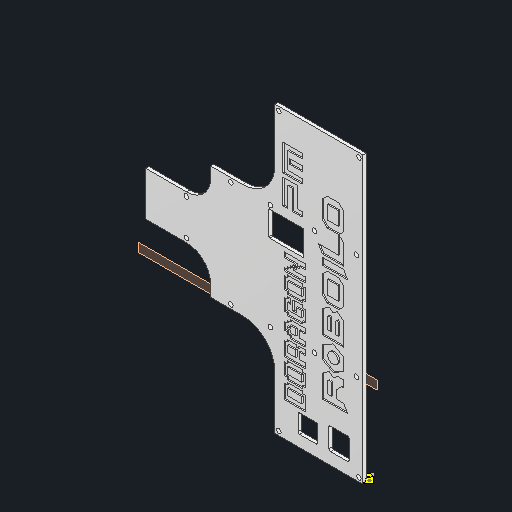
# Autodesk Inventor part: ceil
Saved by Autodesk Inventor 2023 (Build 270158000, 158)
## iProperties
Created: 2024-05-26
Part Number: ceil
Material: ABS Plastic
Document SubType Name: Modeling
Designer: szymo
Density: 1.06 g/cm^3
Appearance: Smooth - White
Mass: 27.4887 g
Surface Area: 302.13 cm^2
Volume: 25.9328 cm^3
TOTAL MASS: 0.0
Author: szymo
Autodesk Inventor part; units mm, degrees
ref_plane "YZ Plane" through (0, 0, 0) normal (1, 0, 0) x (0, 1, 0)
ref_plane "XZ Plane" through (0, 0, 0) normal (0, 1, 0) x (-1, 0, 0)
ref_plane "XY Plane" through (0, 0, 0) normal (0, 0, 1) x (1, 0, 0)
ref_plane "Work Plane1" through (-50.5, 0, 0) normal (0, 0, 1) x (1, 0, 0)
sketch "Sketch3" plane through (-50.5, 0, 0) normal (0, 0, 1) x (1, 0, 0)
  line L0 (135.5648, 0) -> (135.5648, 5.2284) projected
  line L1 (0, 5) -> (134.493, 5) projected
  line L2 (0, 0) -> (0, 5) projected
  line L3 (0, 71) -> (135.5648, 71) projected
  line L4 (0, 71) -> (0, 66) projected
  line L5 (0, 66) -> (135.5648, 66) projected
  line L6 (135.5648, 71) -> (135.5648, 66) projected
  line L7 (131.5648, 119.5) -> (134.5648, 119.5) projected
  line L8 (135.5648, 124.5) -> (135.5648, 120.5) projected
  line L9 (135.5648, 124.5) -> (51.5, 124.5) projected
  line L10 (51.5, 123.5) -> (79.5, 123.5) projected
  line L11 (80.5, 122.5) -> (80.5, 120.5) projected
  line L12 (81.5, 119.5) -> (84.5, 119.5) projected
  line L13 (85.5, 122.5) -> (85.5, 120.5) projected
  line L14 (86.5, 123.5) -> (129.5648, 123.5) projected
  line L15 (130.5648, 122.5) -> (130.5648, 120.5) projected
  line L16 (120.8148, 112) -> (120.8148, 123) projected
  line L17 (120.8148, 123) -> (94.8148, 123) projected
  line L18 (94.8148, 123) -> (94.8148, 112) projected
  line L19 (94.8148, 112) -> (120.8148, 112) projected
  line L20 (130.5648, -51.5) -> (130.5648, -49.5) projected
  line L21 (51.5, -52.5) -> (79.5, -52.5) projected
  line L22 (85.5, -51.5) -> (85.5, -49.5) projected
  line L23 (131.5648, -48.5) -> (134.5648, -48.5) projected
  line L24 (80.5, -51.5) -> (80.5, -49.5) projected
  line L25 (86.5, -52.5) -> (129.5648, -52.5) projected
  line L26 (135.5648, -53.5) -> (51.5, -53.5) projected
  line L27 (135.5648, -53.5) -> (135.5648, -49.5) projected
  line L28 (81.5, -48.5) -> (84.5, -48.5) projected
  line L29 (95.5648, -45.8) -> (95.5648, -35.2) projected
  line L30 (106.8648, -35.2) -> (95.5648, -35.2) projected
  line L31 (106.8648, -35.2) -> (106.8648, -45.8) projected
  line L32 (95.5648, -45.8) -> (106.8648, -45.8) projected
  circle A0 centre (90.4898, -49.075) radius 1.675 projected
  circle A1 centre (124.5398, -49.075) radius 1.675 projected
  line L33 (126.3648, -33.5) -> (126.3648, -45.5) projected
  line L34 (126.3648, -45.5) -> (114.7648, -45.5) projected
  line L35 (114.7648, -45.5) -> (114.7648, -33.5) projected
  line L36 (114.7648, -33.5) -> (86.8648, -33.5) projected
  line L37 (86.8648, -33.5) -> (86.8648, -52.5) projected
  line L38 (86.8648, -52.5) -> (128.0648, -52.5) projected
  line L39 (128.0648, -52.5) -> (128.0648, -33.5) projected
  line L40 (128.0648, -33.5) -> (126.3648, -33.5) projected
  line L41 (126.3648, -32.7) -> (114.7648, -32.7) projected
  line L42 (114.7648, -32.7) -> (114.7648, -45.5) projected
  line L43 (114.7648, -45.5) -> (126.3648, -45.5) projected
  line L44 (126.3648, -45.5) -> (126.3648, -32.7) projected
  line L45 (80.5, -53.5) -> (135.5648, -53.5)
  line L46 (135.5648, -53.5) -> (135.5648, 124.5)
  line L47 (135.5648, 124.5) -> (80.5, 124.5)
  line L48 (80.5, 124.5) -> (80.5, -53.5)
  line L49 (0, 22) -> (80.5, 22)
  line L50 (80.5, 22) -> (80.5, 49.5)
  line L51 (80.5, 49.5) -> (0, 49.5)
  line L52 (0, 49.5) -> (0, 22)
  line L53 (80.5, 22) -> (50.5, 22)
  line L54 (50.5, 22) -> (50.5, 0)
  line L55 (50.5, 0) -> (80.5, 0)
  line L56 (80.5, 0) -> (80.5, 22)
  line L57 (80.5, 46.5815) -> (80.5, 71)
  line L58 (80.5, 71) -> (50.5, 71)
  line L59 (50.5, 71) -> (50.5, 49.5)
  arc A2 (97.9124, 50.9) -> (98.0124, 51) centre (97.9124, 51) ccw projected
  line L60 (77.4124, 50.9) -> (97.9124, 50.9) projected
  arc A3 (77.3124, 51) -> (77.4124, 50.9) centre (77.4124, 51) ccw projected
  line L61 (77.3124, 65.5) -> (77.3124, 51) projected
  arc A4 (77.4124, 65.6) -> (77.3124, 65.5) centre (77.4124, 65.5) ccw projected
  line L62 (97.9124, 65.6) -> (77.4124, 65.6) projected
  arc A5 (98.0124, 65.5) -> (97.9124, 65.6) centre (97.9124, 65.5) ccw projected
  line L63 (98.0124, 51) -> (98.0124, 65.5) projected
  line L64 (96.2124, 63.7) -> (96.2124, 52.8) projected
  arc A6 (96.2124, 63.7) -> (95.9124, 64) centre (95.9124, 63.7) ccw projected
  line L65 (95.9124, 64) -> (95.8124, 64) projected
  line L66 (95.8124, 64) -> (95.3509, 64.55) projected
  line L67 (95.3509, 64.55) -> (94.9739, 64.55) projected
  line L68 (94.9739, 64.55) -> (94.5124, 64) projected
  line L69 (94.5124, 64) -> (90.8124, 64) projected
  line L70 (90.8124, 64) -> (90.8124, 64.35) projected
  line L71 (90.8124, 64.35) -> (89.5124, 64.35) projected
  line L72 (89.5124, 64) -> (89.5124, 64.35) projected
  line L73 (89.5124, 64) -> (85.8124, 64) projected
  line L74 (85.8124, 64) -> (85.8124, 64.35) projected
  line L75 (85.8124, 64.35) -> (84.5124, 64.35) projected
  line L76 (84.5124, 64) -> (84.5124, 64.35) projected
  line L77 (84.5124, 64) -> (80.8124, 64) projected
  line L78 (80.8124, 64) -> (80.3509, 64.55) projected
  line L79 (80.3509, 64.55) -> (79.9739, 64.55) projected
  line L80 (79.9739, 64.55) -> (79.5124, 64) projected
  line L81 (79.5124, 64) -> (79.4124, 64) projected
  arc A7 (79.4124, 64) -> (79.1124, 63.7) centre (79.4124, 63.7) ccw projected
  line L82 (79.1124, 63.7) -> (79.1124, 52.8) projected
  arc A8 (79.1124, 52.8) -> (79.4124, 52.5) centre (79.4124, 52.8) ccw projected
  line L83 (79.4124, 52.5) -> (79.5124, 52.5) projected
  line L84 (79.5124, 52.5) -> (79.9739, 51.95) projected
  line L85 (80.3509, 51.95) -> (79.9739, 51.95) projected
  line L86 (80.3509, 51.95) -> (80.8124, 52.5) projected
  line L87 (80.8124, 52.5) -> (84.5124, 52.5) projected
  line L88 (84.5124, 52.5) -> (84.5124, 52.15) projected
  line L89 (85.8124, 52.15) -> (84.5124, 52.15) projected
  line L90 (85.8124, 52.5) -> (85.8124, 52.15) projected
  line L91 (85.8124, 52.5) -> (89.5124, 52.5) projected
  line L92 (89.5124, 52.5) -> (89.5124, 52.15) projected
  line L93 (90.8124, 52.15) -> (89.5124, 52.15) projected
  line L94 (90.8124, 52.5) -> (90.8124, 52.15) projected
  line L95 (90.8124, 52.5) -> (94.5124, 52.5) projected
  line L96 (94.5124, 52.5) -> (94.9739, 51.95) projected
  line L97 (95.3509, 51.95) -> (94.9739, 51.95) projected
  line L98 (95.3509, 51.95) -> (95.8124, 52.5) projected
  line L99 (95.8124, 52.5) -> (95.9124, 52.5) projected
  arc A9 (95.9124, 52.5) -> (96.2124, 52.8) centre (95.9124, 52.8) ccw projected
  line L100 (78.1624, 55.35) -> (78.8624, 55.35) projected
  line L101 (78.8624, 55.35) -> (78.8624, 61.15) projected
  line L102 (78.1624, 61.15) -> (78.8624, 61.15) projected
  line L103 (78.1624, 61.15) -> (78.1624, 55.35) projected
  line L104 (97.1624, 61.15) -> (97.1624, 55.35) projected
  line L105 (96.4624, 61.15) -> (97.1624, 61.15) projected
  line L106 (96.4624, 55.35) -> (96.4624, 61.15) projected
  line L107 (96.4624, 55.35) -> (97.1624, 55.35) projected
  arc A10 (76.8124, 51) -> (77.4124, 50.4) centre (77.4124, 51) ccw
  line L108 (77.4124, 50.4) -> (97.9124, 50.4)
  arc A11 (97.9124, 50.4) -> (98.5124, 51) centre (97.9124, 51) ccw
  line L109 (98.5124, 51) -> (98.5124, 65.5)
  arc A12 (98.5124, 65.5) -> (97.9124, 66.1) centre (97.9124, 65.5) ccw
  line L110 (97.9124, 66.1) -> (77.4124, 66.1)
  arc A13 (77.4124, 66.1) -> (76.8124, 65.5) centre (77.4124, 65.5) ccw
  line L111 (76.8124, 65.5) -> (76.8124, 51)
  line L112 (95.0648, -34.7) -> (95.0648, -46.3)
  line L113 (95.0648, -46.3) -> (107.3648, -46.3)
  line L114 (107.3648, -46.3) -> (107.3648, -34.7)
  line L115 (107.3648, -34.7) -> (95.0648, -34.7)
  line L116 (114.2648, -45.5) -> (114.2648, -32.2)
  line L117 (114.2648, -32.2) -> (126.8648, -32.2)
  line L118 (126.8648, -32.2) -> (126.8648, -45.5)
  line L119 (126.3648, -46) -> (114.7648, -46)
  line L120 (92.8148, 110) -> (92.8148, 125)
  line L121 (92.8148, 125) -> (122.8148, 125)
  line L122 (122.8148, 125) -> (122.8148, 110)
  line L123 (122.8148, 110) -> (92.8148, 110)
  line L124 (114.2648, -45.5) -> (114.2648, -46)
  line L125 (114.2648, -46) -> (114.7648, -46)
  line L126 (126.3648, -46) -> (126.8648, -46)
  line L127 (126.8648, -46) -> (126.8648, -45.5)
  line L128 (51.5, -53.5) -> (51.5, -52.5) projected
  line L129 (51.5, 124.5) -> (51.5, 123.5) projected
  circle A14 centre (105.3205, 68.5) radius 1.75 projected
  circle A15 centre (53, 68.5) radius 1.75 projected
  circle A16 centre (77.648, 2.5) radius 1.75 projected
  circle A17 centre (131.5519, 2.5) radius 1.75 projected
  circle A18 centre (83, 122) radius 1.75 projected
  circle A19 centre (133.0648, 122) radius 1.75 projected
  arc A20 (130.5648, 120.5) -> (131.5648, 119.5) centre (131.5648, 120.5) ccw projected
  arc A21 (134.5648, 119.5) -> (135.5648, 120.5) centre (134.5648, 120.5) ccw projected
  arc A22 (80.5, 122.5) -> (79.5, 123.5) centre (79.5, 122.5) ccw projected
  arc A23 (86.5, 123.5) -> (85.5, 122.5) centre (86.5, 122.5) ccw projected
  arc A24 (130.5648, 122.5) -> (129.5648, 123.5) centre (129.5648, 122.5) ccw projected
  arc A25 (80.5, 120.5) -> (81.5, 119.5) centre (81.5, 120.5) ccw projected
  arc A26 (84.5, 119.5) -> (85.5, 120.5) centre (84.5, 120.5) ccw projected
  circle A27 centre (83, -51) radius 1.75 projected
  circle A28 centre (133.0648, -51) radius 1.75 projected
  arc A29 (131.5648, -48.5) -> (130.5648, -49.5) centre (131.5648, -49.5) ccw projected
  arc A30 (129.5648, -52.5) -> (130.5648, -51.5) centre (129.5648, -51.5) ccw projected
  arc A31 (85.5, -51.5) -> (86.5, -52.5) centre (86.5, -51.5) ccw projected
  arc A32 (79.5, -52.5) -> (80.5, -51.5) centre (79.5, -51.5) ccw projected
  arc A33 (135.5648, -49.5) -> (134.5648, -48.5) centre (134.5648, -49.5) ccw projected
  arc A34 (85.5, -49.5) -> (84.5, -48.5) centre (84.5, -49.5) ccw projected
  arc A35 (81.5, -48.5) -> (80.5, -49.5) centre (81.5, -49.5) ccw projected
  line L130 (50.5, 27) -> (0, 27) projected
  line L131 (0, 27) -> (0, 22) projected
  line L132 (50.5, 22) -> (0, 22) projected
  line L133 (50.5, 27) -> (50.5, 22) projected
  line L134 (50.5, 44.5) -> (0, 44.5) projected
  line L135 (50.5, 44.5) -> (50.5, 49.5) projected
  line L136 (50.5, 49.5) -> (0, 49.5) projected
  line L137 (0, 44.5) -> (0, 49.5) projected
  line L138 (50.5, 0) -> (40.5, 0)
  line L139 (40.5, 0) -> (40.5, 22)
  line L140 (40.5, 22) -> (50.5, 22)
  line L141 (50.5, 22) -> (50.5, 0)
  line L142 (50.5, 49.5) -> (40.5, 49.5)
  line L143 (40.5, 49.5) -> (40.5, 71)
  line L144 (40.5, 71) -> (50.5, 71)
  line L145 (50.5, 71) -> (50.5, 49.5)
  ellipse E0 centre (134.493, 7) end of major axis (136.8024, 7) minor radius 2 (134.493, 5) -> (135.5648, 5.2284) ccw projected
  circle A36 centre (25.25, 47) radius 1.75 projected
  circle A37 centre (25.25, 24.5) radius 1.75 projected
  line L146 (0, 0) -> (3.5, 0) projected
  line L147 (3.5, 0) -> (47, 0) projected
  line L148 (47, 0) -> (135.5648, 0) projected
  circle A38 centre (105.3205, 2.5) radius 1.75 projected
  circle A39 centre (53, 2.5) radius 1.75 projected
  point P0 (80.5, -49.5)
  point P1 (80.5, -52.5)
  point P2 (122.8148, 124.5)
  point P3 (92.8148, 124.5)
  point P4 (0, 44)
  point P5 (50.5, 44)
  point P6 (122.8148, 124.5)
  point P7 (122.8148, 123.5)
  point P8 (92.8148, 123.5)
  point P9 (92.8148, 124.5)
  point P10 (80.5, 123.5)
  point P11 (50.5, 66)
  point P12 (50.5, 5)
  point P13 (80.5, -52.5)
  point P14 (80.5, 66)
  point P15 (80.5, 5)
  point P16 (135.5648, 5)
  point P17 (80.5, 22)
  point P18 (50.5, 27)
  point P19 (0, 27)
  point P20 (135.5648, -49.5)
  point P21 (80.5, -49.5)
  point P22 (77.0807, 66)
  point P23 (80.5, 66.1)
  point P24 (135.5648, 5.2284)
  point P25 (80.5, 50.4)
  point P26 (40.5, 5)
  dimension "d16" = 0.5
  dimension "d17" = 0.5
  dimension "d18" = 0.5
  dimension "d19" = 0.5
  dimension "d20" = 2
  dimension "d191" = 10
  dimension "d192" = 10
  constraints: 84 end point, 11 parallel, 8 point on circle, 7 perpendicular, 6 horizontal, 5 point on line, 4 centre point, 4 vertical, 1 collinear, 22 other
  measures "d16" distance between parallel lines of L61 L111
  measures "d17" distance between parallel lines of L29 L112
  measures "d18" distance between parallel lines of L42 L116
  measures "d19" distance between parallel lines of L34 L119
  measures "d20" distance between parallel lines of L18 L120
  measures "d191" distance between parallel lines of L139 L54
  measures "d192" distance between parallel lines of L59 L143
extrude "Extrusion2" add sketch "Sketch3" along normal blind 2 contours L148 L48 L1 E0 L0 | L46 A33 L23 A29 L20 A30 L25 L39 L40 L118 L117 L116 L36 L37 A31 L22 A34 L28 A35 L48 L148 | E0 L1 L48 L108 A11 L109 A12 L5 L46 | L27 L26 L48 L24 A35 L28 A34 L22 A31 L25 A30 L20 A29 L23 A33 | L55 L54 L1 L48 | L5 A12 L110 L48 L3 L6 | L1 L54 L49 L48 | L138 L139 L1 L54 | L3 L48 A25 L12 A26 L13 A23 L14 L120 L123 L122 A24 L15 A20 L7 A21 L46 | L1 L139 L49 L54 | L49 L133 L130 L52 L134 L135 L51 L48 | L5 A13 L110 L48 | L48 L110 A13 L5 L59 L3 | A21 L7 A20 L15 A24 L14 L122 L9 L8 | L49 L52 L130 L133 | A13 L111 A10 L108 L48 L51 L59 L5 | L59 L5 L143 L3 | L11 L48 L9 L120 L14 A23 L13 A26 L12 A25 | L59 L51 L143 L5 | L122 L14 L120 L9 | L135 L134 L52 L51 | L122 L123 L120 L14 | L25 L37 L36 L116 L124 L125 L119 L126 L127 L118 L40 L39 | L19 L18 L17 L16 | A0 | A1 | A14 | A15 | A16 | A17 | A18 | A19 | A27 | A28 | A36 | A37 | A38 | A39
fillet "Fillet2" radius 1 8 edges at (44.5648, -46.3, 1) (44.5648, -34.7, 1) (56.8648, -34.7, 1) (56.8648, -46.3, 1) (63.7648, -46, 1) (63.7648, -32.2, 1) (76.3648, -32.2, 1) (76.3648, -46, 1)
fillet "Fillet3" radius 20 2 edges at (30, 71, 1) (30, 0, 1)
sketch "Sketch4" plane through (-50.5, 0, 2) normal (0, 0, 1) x (1, 0, 0)
  line L0 (130.5648, -51.5) -> (130.5648, -49.5) projected
  line L1 (51.5, -52.5) -> (79.5, -52.5) projected
  line L2 (85.5, -51.5) -> (85.5, -49.5) projected
  line L3 (131.5648, -48.5) -> (134.5648, -48.5) projected
  line L4 (80.5, -51.5) -> (80.5, -49.5) projected
  line L5 (86.5, -52.5) -> (129.5648, -52.5) projected
  line L6 (135.5648, -53.5) -> (51.5, -53.5) projected
  line L7 (135.5648, -53.5) -> (135.5648, -49.5) projected
  line L8 (81.5, -48.5) -> (84.5, -48.5) projected
  line L9 (131.5648, 119.5) -> (134.5648, 119.5) projected
  line L10 (135.5648, 124.5) -> (135.5648, 120.5) projected
  line L11 (135.5648, 124.5) -> (51.5, 124.5) projected
  line L12 (51.5, 123.5) -> (79.5, 123.5) projected
  line L13 (80.5, 122.5) -> (80.5, 120.5) projected
  line L14 (81.5, 119.5) -> (84.5, 119.5) projected
  line L15 (85.5, 122.5) -> (85.5, 120.5) projected
  line L16 (86.5, 123.5) -> (129.5648, 123.5) projected
  line L17 (130.5648, 122.5) -> (130.5648, 120.5) projected
  line L18 (51.5, 124.5) -> (51.5, 123.5) projected
  line L19 (51.5, -53.5) -> (51.5, -52.5) projected
  circle A0 centre (83, -51) radius 1.75 projected
  circle A1 centre (133.0648, -51) radius 1.75 projected
  arc A2 (131.5648, -48.5) -> (130.5648, -49.5) centre (131.5648, -49.5) ccw projected
  arc A3 (129.5648, -52.5) -> (130.5648, -51.5) centre (129.5648, -51.5) ccw projected
  arc A4 (85.5, -51.5) -> (86.5, -52.5) centre (86.5, -51.5) ccw projected
  arc A5 (79.5, -52.5) -> (80.5, -51.5) centre (79.5, -51.5) ccw projected
  arc A6 (135.5648, -49.5) -> (134.5648, -48.5) centre (134.5648, -49.5) ccw projected
  arc A7 (85.5, -49.5) -> (84.5, -48.5) centre (84.5, -49.5) ccw projected
  arc A8 (81.5, -48.5) -> (80.5, -49.5) centre (81.5, -49.5) ccw projected
  circle A9 centre (83, 122) radius 1.75 projected
  circle A10 centre (133.0648, 122) radius 1.75 projected
  arc A11 (130.5648, 120.5) -> (131.5648, 119.5) centre (131.5648, 120.5) ccw projected
  arc A12 (134.5648, 119.5) -> (135.5648, 120.5) centre (134.5648, 120.5) ccw projected
  arc A13 (80.5, 122.5) -> (79.5, 123.5) centre (79.5, 122.5) ccw projected
  arc A14 (86.5, 123.5) -> (85.5, 122.5) centre (86.5, 122.5) ccw projected
  arc A15 (130.5648, 122.5) -> (129.5648, 123.5) centre (129.5648, 122.5) ccw projected
  arc A16 (80.5, 120.5) -> (81.5, 119.5) centre (81.5, 120.5) ccw projected
  arc A17 (84.5, 119.5) -> (85.5, 120.5) centre (84.5, 120.5) ccw projected
  line L20 (50.5, 27) -> (0, 27) projected
  line L21 (0, 27) -> (0, 22) projected
  line L22 (50.5, 22) -> (0, 22) projected
  line L23 (50.5, 27) -> (50.5, 22) projected
  line L24 (50.5, 44.5) -> (0, 44.5) projected
  line L25 (50.5, 44.5) -> (50.5, 49.5) projected
  line L26 (50.5, 49.5) -> (0, 49.5) projected
  line L27 (0, 44.5) -> (0, 49.5) projected
  circle A18 centre (77.648, 68.5) radius 1.75 projected
  circle A19 centre (105.3205, 68.5) radius 1.75 projected
  circle A20 centre (53, 68.5) radius 1.75 projected
  circle A21 centre (131.5519, 68.5) radius 1.75 projected
  line L28 (0, 71) -> (0, 66) projected
  line L29 (0, 66) -> (134.493, 66) projected
  line L30 (135.5648, 71) -> (135.5648, 65.7716) projected
  circle A22 centre (77.648, 2.5) radius 1.75 projected
  circle A23 centre (105.3205, 2.5) radius 1.75 projected
  circle A24 centre (53, 2.5) radius 1.75 projected
  circle A25 centre (131.5519, 2.5) radius 1.75 projected
  line L31 (135.5648, 0) -> (135.5648, 5.2284) projected
  line L32 (0, 5) -> (134.493, 5) projected
  line L33 (0, 0) -> (0, 5) projected
  ellipse E0 centre (134.493, 64) end of major axis (136.8024, 64) minor radius 2 (135.5648, 65.7716) -> (134.493, 66) ccw projected
  ellipse E1 centre (134.493, 7) end of major axis (136.8024, 7) minor radius 2 (134.493, 5) -> (135.5648, 5.2284) ccw projected
  circle A26 centre (25.25, 47) radius 1.75 projected
  circle A27 centre (25.25, 24.5) radius 1.75 projected
  line L34 (0, 71) -> (3.5, 71) projected
  line L35 (47, 71) -> (135.5648, 71) projected
  line L36 (3.5, 71) -> (47, 71) projected
  line L37 (0, 0) -> (3.5, 0) projected
  line L38 (3.5, 0) -> (47, 0) projected
  line L39 (47, 0) -> (135.5648, 0) projected
  point P0 (50.5, 0)
  point P1 (0, 44)
  point P2 (50.5, 44)
  point P3 (50.5, 27)
  point P4 (0, 27)
  constraints: 14 coincident, 2 other
hole "Hole2" at (32.5, -51, 2) at (82.5648, -51, 2) at (82.5648, 122, 2) at (32.5, 122, 2) at (54.8205, 68.5, 2) at (2.5, 2.5, 2) at (2.5, 68.5, 2) at (54.8205, 2.5, 2) at (81.0519, 2.5, 2) at (81.0519, 68.5, 2) at (27.148, 68.5, 2) at (27.148, 2.5, 2) at (-25.25, 24.5, 2) at (-25.25, 47, 2) direction (0, 0, -1) diameter 2.9 end through all clearance for "Countersunk Flat Head Screw ISO 2009/7046" size "M2.5" standard "ISO"
fillet "Fillet4" radius 15 2 edges at (-10, 22, 1) (-10, 49.5, 1)
sketch "Sketch5" plane through (-50.5, 0, 2) normal (0, 0, 1) x (1, 0, 0)
  line L0 (80.5, -53.5) -> (135.5648, -53.5) projected
  line L1 (135.5648, -53.5) -> (135.5648, 124.5) projected
  line L2 (135.5648, 124.5) -> (80.5, 124.5) projected
  line L3 (60.5, 71) -> (40.5, 71) projected
  line L4 (25.5, 49.5) -> (0, 49.5) projected
  line L5 (0, 49.5) -> (0, 22) projected
  line L6 (0, 22) -> (25.5, 22) projected
  line L7 (80.5, 66.1) -> (97.9124, 66.1) projected
  line L8 (97.9124, 50.4) -> (77.4124, 50.4) projected
  arc A0 (76.8124, 51) -> (77.4124, 50.4) centre (77.4124, 51) ccw projected
  line L9 (76.8124, 51) -> (76.8124, 65.5) projected
  arc A1 (77.0807, 66) -> (76.8124, 65.5) centre (77.4124, 65.5) ccw projected
  line L10 (114.2648, -45) -> (114.2648, -33.2) projected
  arc A2 (115.2648, -32.2) -> (114.2648, -33.2) centre (115.2648, -33.2) ccw projected
  line L11 (115.2648, -32.2) -> (125.8648, -32.2) projected
  arc A3 (126.8648, -33.2) -> (125.8648, -32.2) centre (125.8648, -33.2) ccw projected
  line L12 (126.8648, -33.2) -> (126.8648, -45) projected
  arc A4 (125.8648, -46) -> (126.8648, -45) centre (125.8648, -45) ccw projected
  line L13 (125.8648, -46) -> (115.2648, -46) projected
  arc A5 (114.2648, -45) -> (115.2648, -46) centre (115.2648, -45) ccw projected
  line L14 (96.0648, -34.7) -> (106.3648, -34.7) projected
  arc A6 (107.3648, -35.7) -> (106.3648, -34.7) centre (106.3648, -35.7) ccw projected
  line L15 (107.3648, -35.7) -> (107.3648, -45.3) projected
  arc A7 (106.3648, -46.3) -> (107.3648, -45.3) centre (106.3648, -45.3) ccw projected
  line L16 (106.3648, -46.3) -> (96.0648, -46.3) projected
  arc A8 (95.0648, -45.3) -> (96.0648, -46.3) centre (96.0648, -45.3) ccw projected
  line L17 (95.0648, -45.3) -> (95.0648, -35.7) projected
  arc A9 (96.0648, -34.7) -> (95.0648, -35.7) centre (96.0648, -35.7) ccw projected
  line L18 (105.3205, -31.7) -> (105.3205, 48.4) construction
  line L19 (105.3205, 48.4) -> (80.5, 48.4) construction
  line L20 (80.5, 48.4) -> (80.5, -31.7) construction
  line L21 (80.5, -31.7) -> (105.3205, -31.7) construction
  line L22 (110.1651, 28.6458) -> (110.1651, 14.5717) projected
  line L23 (119.2148, -10.52) -> (122.2141, -7.4431) projected
  line L24 (122.2141, -7.4431) -> (123.5648, -7.4431) projected
  line L25 (123.5648, -7.4431) -> (123.5648, -3.1151) projected
  line L26 (123.5648, -3.1151) -> (119.5551, -3.1151) projected
  line L27 (119.5551, -3.1151) -> (117.3584, -5.3021) projected
  line L28 (117.3584, -5.3021) -> (114.3535, -3.0659) projected
  line L29 (114.3535, -3.0659) -> (110.1651, -6.1782) projected
  line L30 (110.1651, -6.1782) -> (110.1651, -20.0711) projected
  line L31 (110.1651, -20.0711) -> (125.9602, -20.0711) projected
  line L32 (125.9602, -20.0711) -> (123.4807, -15.7431) projected
  line L33 (123.4807, -15.7431) -> (119.2148, -15.7431) projected
  line L34 (119.2148, -15.7431) -> (119.2148, -10.52) projected
  line L35 (114.6271, -7.6036) -> (115.8612, -8.5098) projected
  line L36 (115.8612, -8.5098) -> (115.8612, -15.7431) projected
  line L37 (115.8612, -15.7431) -> (113.4584, -15.7431) projected
  line L38 (113.4584, -15.7431) -> (113.4584, -8.4973) projected
  line L39 (113.4584, -8.4973) -> (114.6271, -7.6036) projected
  line L40 (123.5648, 1.4254) -> (123.5648, 9.1617) projected
  line L41 (123.5648, 9.1617) -> (116.8649, 13.0299) projected
  line L42 (116.8649, 13.0299) -> (110.1651, 9.1617) projected
  line L43 (110.1651, 9.1617) -> (110.1651, 1.4254) projected
  line L44 (110.1651, 1.4254) -> (116.8649, -2.4427) projected
  line L45 (116.8649, -2.4427) -> (123.5648, 1.4254) projected
  circle A10 centre (116.8649, 5.2936) radius 3.3 projected
  line L46 (123.5848, 14.5717) -> (123.5848, 28.6458) projected
  line L47 (123.5848, 28.6458) -> (119.3867, 31.747) projected
  line L48 (119.3867, 31.747) -> (116.875, 29.8983) projected
  line L49 (116.875, 29.8983) -> (114.3632, 31.747) projected
  line L50 (114.3632, 31.747) -> (110.1651, 28.6458) projected
  line L51 (110.1651, 28.6458) -> (110.1651, 14.5717) projected
  line L52 (110.1651, 14.5717) -> (123.5848, 14.5717) projected
  line L53 (115.3489, 26.1486) -> (115.3489, 18.8997) projected
  line L54 (115.3489, 18.8997) -> (113.4785, 18.8997) projected
  line L55 (113.4785, 18.8997) -> (113.4785, 26.1539) projected
  line L56 (113.4785, 26.1539) -> (114.3691, 26.9374) projected
  line L57 (114.3691, 26.9374) -> (115.3489, 26.1486) projected
  line L58 (118.4011, 18.8997) -> (118.4011, 26.1486) projected
  line L59 (118.4011, 26.1486) -> (119.3808, 26.9374) projected
  line L60 (119.3808, 26.9374) -> (120.2715, 26.1539) projected
  line L61 (120.2715, 26.1539) -> (120.2715, 18.8997) projected
  line L62 (120.2715, 18.8997) -> (118.4011, 18.8997) projected
  line L63 (120.494, 33.3579) -> (123.5648, 36.4286) projected
  line L64 (123.5648, 36.4286) -> (123.5648, 47.4441) projected
  line L65 (123.5648, 47.4441) -> (120.494, 50.5148) projected
  line L66 (120.494, 50.5148) -> (113.2358, 50.5148) projected
  line L67 (113.2358, 50.5148) -> (110.1651, 47.4441) projected
  line L68 (110.1651, 47.4441) -> (110.1651, 36.4286) projected
  line L69 (110.1651, 36.4286) -> (113.2358, 33.3579) projected
  line L70 (113.2358, 33.3579) -> (120.494, 33.3579) projected
  line L71 (120.2715, 37.686) -> (113.4584, 37.686) projected
  line L72 (113.4584, 37.686) -> (113.4584, 46.1868) projected
  line L73 (113.4584, 46.1868) -> (120.2715, 46.1868) projected
  line L74 (120.2715, 46.1868) -> (120.2715, 37.686) projected
  line L75 (125.9586, 52.2145) -> (123.5013, 56.5425) projected
  line L76 (123.5013, 56.5425) -> (110.1651, 56.5425) projected
  line L77 (110.1651, 56.5425) -> (110.1651, 52.2145) projected
  line L78 (110.1651, 52.2145) -> (125.9586, 52.2145) projected
  line L79 (123.5648, 88.0003) -> (120.494, 91.071) projected
  line L80 (120.494, 91.071) -> (113.2358, 91.071) projected
  line L81 (113.2358, 91.071) -> (110.1651, 88.0003) projected
  line L82 (110.1651, 88.0003) -> (110.1651, 76.9848) projected
  line L83 (110.1651, 76.9848) -> (113.2358, 73.9141) projected
  line L84 (113.2358, 73.9141) -> (120.2715, 73.9141) projected
  line L85 (120.2715, 73.9141) -> (120.2715, 62.7008) projected
  line L86 (120.2715, 62.7008) -> (107.738, 62.7008) projected
  line L87 (107.738, 62.7008) -> (110.2396, 58.3727) projected
  line L88 (110.2396, 58.3727) -> (123.5848, 58.3727) projected
  line L89 (123.5848, 58.3727) -> (123.5848, 70.8415) projected
  line L90 (123.5848, 70.8415) -> (120.5032, 73.9232) projected
  line L91 (120.5032, 73.9232) -> (123.5648, 76.9848) projected
  line L92 (123.5648, 76.9848) -> (123.5648, 88.0003) projected
  line L93 (120.2715, 78.2421) -> (113.4584, 78.2421) projected
  line L94 (113.4584, 78.2421) -> (113.4584, 86.743) projected
  line L95 (113.4584, 86.743) -> (120.2715, 86.743) projected
  line L96 (120.2715, 86.743) -> (120.2715, 78.2421) projected
  line L97 (91.5024, 71.975) -> (97.5262, 71.975) projected
  line L98 (97.5262, 71.975) -> (97.5262, 74.9242) projected
  line L99 (97.5262, 74.9242) -> (94.45, 74.9242) projected
  line L100 (94.45, 74.9242) -> (94.45, 87.525) projected
  line L101 (94.45, 87.525) -> (85.5, 87.525) projected
  line L102 (85.5, 87.525) -> (85.5, 71.975) projected
  line L103 (85.5, 71.975) -> (88.675, 71.975) projected
  line L104 (88.675, 71.975) -> (88.675, 84.4887) projected
  line L105 (88.675, 84.4887) -> (91.5024, 84.4887) projected
  line L106 (91.5024, 84.4887) -> (91.5024, 71.975) projected
  line L107 (85.5, 106.5) -> (85.5, 89.825) projected
  line L108 (85.5, 89.825) -> (97.6, 89.825) projected
  line L109 (97.6, 89.825) -> (97.6, 92.775) projected
  line L110 (97.6, 92.775) -> (88.6, 92.775) projected
  line L111 (88.6, 92.775) -> (88.6, 103.4705) projected
  line L112 (88.6, 103.4705) -> (97.5254, 103.4705) projected
  line L113 (97.5254, 103.4705) -> (97.5254, 106.5) projected
  line L114 (97.5254, 106.5) -> (85.5, 106.5) projected
  line L115 (89.7, 99.675) -> (89.7, 96.575) projected
  line L116 (89.7, 96.575) -> (97.6, 96.575) projected
  line L117 (97.6, 96.575) -> (97.6, 99.675) projected
  line L118 (97.6, 99.675) -> (89.7, 99.675) projected
  line L119 (80.5, -20) -> (80.5, -53.5) projected
  line L120 (80.5, 66) -> (80.5, 66.1) projected
  arc A11 (60.5, 71) -> (80.5, 91) centre (60.5, 91) ccw projected
  circle A12 centre (105.3205, 2.5) radius 1.45 projected
  line L121 (40.5, 71) -> (40.5, 64.5) projected
  line L122 (40.5, 7) -> (40.5, 0) projected
  arc A13 (25.5, 49.5) -> (40.5, 64.5) centre (25.5, 64.5) ccw projected
  arc A14 (40.5, 7) -> (25.5, 22) centre (25.5, 7) ccw projected
  line L123 (40.5, 0) -> (60.5, 0) projected
  arc A15 (98.5124, 65.5) -> (97.9124, 66.1) centre (97.9124, 65.5) ccw projected
  line L124 (98.5124, 65.5) -> (98.5124, 51) projected
  arc A16 (97.9124, 50.4) -> (98.5124, 51) centre (97.9124, 51) ccw projected
  line L125 (77.0807, 66) -> (80.5, 66) projected
  line L126 (80.5, 124.5) -> (80.5, 91) projected
  arc A17 (80.5, -20) -> (60.5, 0) centre (60.5, -20) ccw projected
  line L127 (99.4102, -32.275) -> (86.4102, -32.275)
  line L128 (86.4102, -32.275) -> (86.4102, -23.4821)
  line L129 (86.4102, -23.4821) -> (88.2317, -23.4821)
  line L130 (88.2317, -23.4821) -> (88.2317, -22.0607)
  line L131 (88.2317, -22.0607) -> (97.5888, -22.0607)
  line L132 (97.5888, -22.0607) -> (97.5888, -23.4821)
  line L133 (97.5888, -23.4821) -> (99.4102, -23.4821)
  line L134 (99.4102, -23.4821) -> (99.4102, -32.275)
  line L135 (97.3317, -25.1679) -> (88.4888, -25.1679)
  line L136 (88.4888, -25.1679) -> (88.4888, -29.1679)
  line L137 (88.4888, -29.1679) -> (97.3317, -29.1679)
  line L138 (97.3317, -29.1679) -> (97.3317, -25.1679)
  line L139 (99.4102, -19.2464) -> (97.5888, -19.2464)
  line L140 (97.5888, -19.2464) -> (97.5888, -20.6679)
  line L141 (97.5888, -20.6679) -> (88.2317, -20.6679)
  line L142 (88.2317, -20.6679) -> (88.2317, -19.2464)
  line L143 (88.2317, -19.2464) -> (86.4102, -19.2464)
  line L144 (86.4102, -19.2464) -> (86.4102, -11.875)
  line L145 (86.4102, -11.875) -> (88.2317, -11.875)
  line L146 (88.2317, -11.875) -> (88.2317, -10.4536)
  line L147 (88.2317, -10.4536) -> (97.5888, -10.4536)
  line L148 (97.5888, -10.4536) -> (97.5888, -11.875)
  line L149 (97.5888, -11.875) -> (99.4102, -11.875)
  line L150 (99.4102, -11.875) -> (99.4102, -19.2464)
  line L151 (97.3317, -13.5607) -> (88.4888, -13.5607)
  line L152 (88.4888, -13.5607) -> (88.4888, -17.5607)
  line L153 (88.4888, -17.5607) -> (97.3317, -17.5607)
  line L154 (97.3317, -17.5607) -> (97.3317, -13.5607)
  line L155 (99.4102, -9.0607) -> (86.4102, -9.0607)
  line L156 (86.4102, -9.0607) -> (86.4102, -0.2679)
  line L157 (86.4102, -0.2679) -> (88.2317, -0.2679)
  line L158 (88.2317, -0.2679) -> (88.2317, 1.1536)
  line L159 (88.2317, 1.1536) -> (93.9531, 1.1536)
  line L160 (93.9531, 1.1536) -> (93.9531, -0.2679)
  line L161 (93.9531, -0.2679) -> (95.5102, -0.2679)
  line L162 (95.5102, -0.2679) -> (95.5102, 1.1536)
  line L163 (95.5102, 1.1536) -> (99.4102, 1.1536)
  line L164 (99.4102, 1.1536) -> (99.4102, -1.9536)
  line L165 (99.4102, -1.9536) -> (95.7674, -1.9536)
  line L166 (95.7674, -1.9536) -> (95.7674, -5.9536)
  line L167 (95.7674, -5.9536) -> (99.4102, -5.9536)
  line L168 (99.4102, -5.9536) -> (99.4102, -9.0607)
  line L169 (93.6959, -1.9536) -> (88.4888, -1.9536)
  line L170 (88.4888, -1.9536) -> (88.4888, -5.9536)
  line L171 (88.4888, -5.9536) -> (93.6959, -5.9536)
  line L172 (93.6959, -5.9536) -> (93.6959, -1.9536)
  line L173 (99.4102, 2.5464) -> (90.0531, 2.5464)
  line L174 (90.0531, 2.5464) -> (90.0531, 3.9679)
  line L175 (90.0531, 3.9679) -> (88.2317, 3.9679)
  line L176 (88.2317, 3.9679) -> (88.2317, 5.3893)
  line L177 (88.2317, 5.3893) -> (86.4102, 5.3893)
  line L178 (86.4102, 5.3893) -> (86.4102, 9.9179)
  line L179 (86.4102, 9.9179) -> (88.2317, 9.9179)
  line L180 (88.2317, 9.9179) -> (88.2317, 11.3393)
  line L181 (88.2317, 11.3393) -> (90.0531, 11.3393)
  line L182 (90.0531, 11.3393) -> (90.0531, 12.7607)
  line L183 (90.0531, 12.7607) -> (99.4102, 12.7607)
  line L184 (99.4102, 12.7607) -> (99.4102, 9.6536)
  line L185 (99.4102, 9.6536) -> (95.7674, 9.6536)
  line L186 (95.7674, 9.6536) -> (95.7674, 5.6536)
  line L187 (95.7674, 5.6536) -> (99.4102, 5.6536)
  line L188 (99.4102, 5.6536) -> (99.4102, 2.5464)
  line L189 (93.6959, 9.6536) -> (90.3102, 9.6536)
  line L190 (90.3102, 9.6536) -> (90.3102, 8.2321)
  line L191 (90.3102, 8.2321) -> (88.4888, 8.2321)
  line L192 (88.4888, 8.2321) -> (88.4888, 7.075)
  line L193 (88.4888, 7.075) -> (90.3102, 7.075)
  line L194 (90.3102, 7.075) -> (90.3102, 5.6536)
  line L195 (90.3102, 5.6536) -> (93.6959, 5.6536)
  line L196 (93.6959, 5.6536) -> (93.6959, 9.6536)
  line L197 (99.4102, 15.575) -> (97.5888, 15.575)
  line L198 (97.5888, 15.575) -> (97.5888, 14.1536)
  line L199 (97.5888, 14.1536) -> (88.2317, 14.1536)
  line L200 (88.2317, 14.1536) -> (88.2317, 15.575)
  line L201 (88.2317, 15.575) -> (86.4102, 15.575)
  line L202 (86.4102, 15.575) -> (86.4102, 22.9464)
  line L203 (86.4102, 22.9464) -> (88.2317, 22.9464)
  line L204 (88.2317, 22.9464) -> (88.2317, 24.3679)
  line L205 (88.2317, 24.3679) -> (90.3102, 24.3679)
  line L206 (90.3102, 24.3679) -> (90.3102, 21.2607)
  line L207 (90.3102, 21.2607) -> (88.4888, 21.2607)
  line L208 (88.4888, 21.2607) -> (88.4888, 17.2607)
  line L209 (88.4888, 17.2607) -> (97.3317, 17.2607)
  line L210 (97.3317, 17.2607) -> (97.3317, 21.2607)
  line L211 (97.3317, 21.2607) -> (93.9531, 21.2607)
  line L212 (93.9531, 21.2607) -> (93.9531, 18.4179)
  line L213 (93.9531, 18.4179) -> (91.8745, 18.4179)
  line L214 (91.8745, 18.4179) -> (91.8745, 24.3679)
  line L215 (91.8745, 24.3679) -> (97.5888, 24.3679)
  line L216 (97.5888, 24.3679) -> (97.5888, 22.9464)
  line L217 (97.5888, 22.9464) -> (99.4102, 22.9464)
  line L218 (99.4102, 22.9464) -> (99.4102, 15.575)
  line L219 (99.4102, 27.1821) -> (97.5888, 27.1821)
  line L220 (97.5888, 27.1821) -> (97.5888, 25.7607)
  line L221 (97.5888, 25.7607) -> (88.2317, 25.7607)
  line L222 (88.2317, 25.7607) -> (88.2317, 27.1821)
  line L223 (88.2317, 27.1821) -> (86.4102, 27.1821)
  line L224 (86.4102, 27.1821) -> (86.4102, 34.5536)
  line L225 (86.4102, 34.5536) -> (88.2317, 34.5536)
  line L226 (88.2317, 34.5536) -> (88.2317, 35.975)
  line L227 (88.2317, 35.975) -> (97.5888, 35.975)
  line L228 (97.5888, 35.975) -> (97.5888, 34.5536)
  line L229 (97.5888, 34.5536) -> (99.4102, 34.5536)
  line L230 (99.4102, 34.5536) -> (99.4102, 27.1821)
  line L231 (97.3317, 32.8679) -> (88.4888, 32.8679)
  line L232 (88.4888, 32.8679) -> (88.4888, 28.8679)
  line L233 (88.4888, 28.8679) -> (97.3317, 28.8679)
  line L234 (97.3317, 28.8679) -> (97.3317, 32.8679)
  line L235 (99.4102, 44.475) -> (95.7674, 44.475)
  line L236 (95.7674, 44.475) -> (95.7674, 43.0536)
  line L237 (95.7674, 43.0536) -> (93.6959, 43.0536)
  line L238 (93.6959, 43.0536) -> (93.6959, 44.475)
  line L239 (93.6959, 44.475) -> (86.4102, 44.475)
  line L240 (86.4102, 44.475) -> (86.4102, 47.5821)
  line L241 (86.4102, 47.5821) -> (99.4102, 47.5821)
  line L242 (99.4102, 47.5821) -> (99.4102, 44.475)
  line L243 (99.4102, 37.3679) -> (86.4102, 37.3679)
  line L244 (86.4102, 37.3679) -> (86.4102, 39.0536)
  line L245 (86.4102, 39.0536) -> (88.2317, 39.0536)
  line L246 (88.2317, 39.0536) -> (88.2317, 40.475)
  line L247 (88.2317, 40.475) -> (90.0531, 40.475)
  line L248 (90.0531, 40.475) -> (90.0531, 41.8964)
  line L249 (90.0531, 41.8964) -> (92.1317, 41.8964)
  line L250 (92.1317, 41.8964) -> (92.1317, 40.475)
  line L251 (92.1317, 40.475) -> (99.4102, 40.475)
  line L252 (99.4102, 40.475) -> (99.4102, 37.3679)
  line L253 (93.9531, 41.6321) -> (91.8745, 41.6321)
  line L254 (91.8745, 41.6321) -> (91.8745, 43.3179)
  line L255 (91.8745, 43.3179) -> (93.9531, 43.3179)
  line L256 (93.9531, 43.3179) -> (93.9531, 41.6321)
  point P0 (50.5, 0)
  point P1 (80.5, -20)
  dimension "d188" = 3
  dimension "d189" = 2
  constraints: 2 point on line, 2 other
  measures "d188" distance between parallel lines of L14 L21
  measures "d189" distance between parallel lines of L8 L19
extrude "Extrusion4" cut sketch "Sketch5" against normal blind 0.8 contours L50 L49 L48 L47 L46 L52 L22 | L34 L33 L32 L31 L30 L29 L28 L27 L26 L25 L24 L23 | L45 L44 L43 L42 L41 L40 | L70 L69 L68 L67 L66 L65 L64 L63 | L78 L77 L76 L75 | L92 L91 L90 L89 L88 L87 L86 L85 L84 L83 L82 L81 L80 L79 | L106 L105 L104 L103 L102 L101 L100 L99 L98 L97 | L114 L113 L112 L111 L110 L109 L108 L107 | L118 L117 L116 L115 | L127 L128 L129 L130 L131 L132 L133 L134 | L139 L140 L141 L142 L143 L144 L145 L146 L147 L148 L149 L150 | L155 L156 L157 L158 L159 L160 L161 L162 L163 L164 L165 L166 L167 L168 | L173 L174 L175 L176 L177 L178 L179 L180 L181 L182 L183 L184 L185 L186 L187 L188 | L197 L198 L199 L200 L201 L202 L203 L204 L205 L206 L207 L208 L209 L210 L211 L212 L213 L214 L215 L216 L217 L218 | L219 L220 L221 L222 L223 L224 L225 L226 L227 L228 L229 L230 | L235 L236 L237 L256 L255 L238 L239 L240 L241 L242 | L256 L253 L250 L249 L254 L255 L238 L237 | L237 L238 L255 L256 | L253 L254 L249 L250 | L250 L251 L252 L243 L244 L245 L246 L247 L248 L249 L254 L253
body "Solid2"
